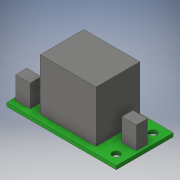
# Autodesk Inventor part: GDT
Saved by Autodesk Inventor 2016 (Build 200138000, 138)
## iProperties
Created: 2018-05-17
Part Number: GDT
Material: Generic
Document SubType Name: Modeling
Designer: Phil Erle
Density: 1 g/cm^3
Appearance: Default
Author: Phil Erle
Autodesk Inventor part; units mm, degrees
ref_plane "YZ Plane" through (0, 0, 0) normal (1, 0, 0) x (0, 1, 0)
ref_plane "XZ Plane" through (0, 0, 0) normal (0, 1, 0) x (-1, 0, 0)
ref_plane "XY Plane" through (0, 0, 0) normal (0, 0, 1) x (1, 0, 0)
sketch "Sketch1" plane through (0, 0, 0) normal (0, 0, 1) x (1, 0, 0)
  line L0 (-24.5, -12.75) -> (24.5, -12.75)
  line L1 (24.5, -12.75) -> (24.5, 12.75)
  line L2 (24.5, 12.75) -> (-24.5, 12.75)
  line L3 (-24.5, 12.75) -> (-24.5, -12.75)
  line L4 (-24.5, -12.75) -> (24.5, 12.75) construction
  line L5 (24.5, -12.75) -> (-24.5, 12.75) construction
  point P0 (0, 0)
  dimension "d0" = 49
  dimension "d1" = 25.5
  constraints: 12 end point, 2 midpoint, 2 parallel, 1 horizontal, 1 perpendicular
  measures "d0" distance of L2.end L1.end
  measures "d1" distance of L0.end L1.end
extrude "Extrusion1" add sketch "Sketch1" along normal blind 1.6
sketch "Sketch2" plane through (0, 0, 1.6) normal (0, 0, 1) x (1, 0, 0)
  line L0 (-12.5, -9.75) -> (12.5, -9.75)
  line L1 (12.5, -9.75) -> (12.5, 9.75)
  line L2 (12.5, 9.75) -> (-12.5, 9.75)
  line L3 (-12.5, 9.75) -> (-12.5, -9.75)
  line L4 (-12.5, -9.75) -> (12.5, 9.75) construction
  line L5 (12.5, -9.75) -> (-12.5, 9.75) construction
  point P0 (0, 0)
  dimension "d4" = 25
  dimension "d5" = 19.5
  constraints: 12 end point, 2 midpoint, 2 parallel, 1 horizontal, 1 perpendicular
  measures "d4" distance of L2.end L1.end
  measures "d5" distance of L0.end L1.end
extrude "Extrusion2" add sketch "Sketch2" along normal blind 23
sketch "Sketch3" plane through (0, 0, 1.6) normal (0, 0, 1) x (1, 0, 0)
  line L0 (16.75, 2.5) -> (23.25, 2.5)
  line L1 (23.25, 2.5) -> (23.25, -2.5)
  line L2 (23.25, -2.5) -> (16.75, -2.5)
  line L3 (16.75, -2.5) -> (16.75, 2.5)
  line L4 (-23.25, 10) -> (-16.75, 10)
  line L5 (-16.75, 10) -> (-16.75, 5)
  line L6 (-16.75, 5) -> (-23.25, 5)
  line L7 (-23.25, 5) -> (-23.25, 10)
  line L8 (-23.25, -5) -> (-16.75, -5)
  line L9 (-16.75, -5) -> (-16.75, -10)
  line L10 (-16.75, -10) -> (-23.25, -10)
  line L11 (-23.25, -10) -> (-23.25, -5)
  line L12 (24.5, -12.75) -> (24.5, 12.75) construction
  line L13 (-16.75, 5) -> (-16.75, -5) construction
  point P0 (0, 0)
  point P1 (23.25, 0)
  point P2 (-16.75, 0)
  dimension "d8" = 5
  dimension "d9" = 5
  dimension "d10" = 5
  dimension "d11" = 6.5
  dimension "d12" = 6.5
  dimension "d13" = 6.5
  dimension "d14" = 33.5
  dimension "d15" = 1.25
  dimension "d16" = 10
  constraints: 26 end point, 6 parallel, 3 horizontal, 3 perpendicular, 2 horizontal alignment, 2 midpoint, 1 vertical alignment
  measures "d8" distance of L6.end L4.start
  measures "d9" distance of L10.end L8.start
  measures "d10" distance of L0.end L1.end
  measures "d11" distance of L0.start L0.end
  measures "d12" distance of L4.start L4.end
  measures "d13" distance of L8.start L8.end
  measures "d14" distance between parallel lines of L3 L5
  measures "d15" distance between parallel lines of L12 L1
  measures "d16" distance of L5.end L8.end
extrude "Extrusion3" add sketch "Sketch3" along normal blind 10
sketch "Sketch4" plane through (0, 0, 1.6) normal (0, 0, 1) x (1, 0, 0)
  line L0 (20, 8.25) -> (20, -8.25) construction
  line L1 (-24.5, 12.75) -> (-24.5, -12.75) projected
  point P0 (0, 0)
  point P1 (-20, 0)
  point P2 (20, 0)
  dimension "d19" = 40
  dimension "d20" = 16.5
  dimension "d21" = 4.5
  constraints: 2 end point, 2 horizontal alignment, 1 midpoint, 1 vertical
  measures "d19" horizontal distance of L0.start point (-20, 0)
  measures "d20" distance of L0.end L0.start
  measures "d21" distance from line of L1 point (-20, 0)
hole "Hole1" at (-20, 0, 1.6) at (20, 8.25, 1.6) at (20, -8.25, 1.6) direction (0, 0, -1) diameter 3.4 depth 8 tip angle 118 clearance for "Countersunk Flat Head Screw DIN EN ISO 2009" size "M3" standard "DIN"
body "Solid1"
